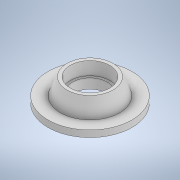
# Autodesk Inventor part: base reaction wheel
Saved by Autodesk Inventor 2021 (Build 250183000, 183)
## iProperties
Created: 2021-07-29
Part Number: base reaction wheel
Material: Generic
Document SubType Name: Modeling
Designer: samlo
Density: 1 g/cm^3
Appearance: Default
Author: samlo
Autodesk Inventor part; units mm, degrees
ref_plane "YZ Plane" through (0, 0, 0) normal (1, 0, 0) x (0, 1, 0)
ref_plane "XZ Plane" through (0, 0, 0) normal (0, 1, 0) x (-1, 0, 0)
ref_plane "XY Plane" through (0, 0, 0) normal (0, 0, 1) x (1, 0, 0)
sketch "Sketch2" plane through (0, 0, 0) normal (0, 0, 1) x (1, 0, 0)
  line L0 (10.49, 0) -> (25.49, 0)
  line L1 (25.49, 0) -> (25.49, 4)
  line L2 (25.49, 4) -> (17.99, 4)
  line L3 (17.99, 4) -> (13.99, 14)
  line L4 (13.99, 14) -> (11.99, 14)
  line L5 (11.99, 14) -> (11.99, 6)
  line L6 (11.99, 6) -> (10.49, 6)
  line L7 (10.49, 6) -> (10.49, 0)
  line L8 (0, -2.8) -> (0, 16.8) projected
  point P0 (0, 0)
  dimension "d0" = 11.99
  dimension "d1" = 1.5
  dimension "d2" = 2
  dimension "d3" = 15
  dimension "d4" = 6
  dimension "d5" = 8
  dimension "d6" = 0
  dimension "d7" = 4
  dimension "d8" = 7.5
  constraints: 16 end point, 4 perpendicular, 2 horizontal, 1 parallel
  measures "d0" distance from line of L5 point (0, 0)
  measures "d1" distance of L5.end L6.end
  measures "d2" distance of L3.end L4.end
  measures "d3" distance of L0.start L0.end
  measures "d4" distance of L6.end L0.start
  measures "d5" distance of L4.end L5.end
  measures "d6" distance from line of point (0, 0) L0
  measures "d7" distance of L0.end L1.end
  measures "d8" distance of L1.end L2.end
revolve "Revolution1" add sketch "Sketch2" angle 360 about axis through (0, -10, 0) along (0, 1, 0)
body "Solid1"
